Autodesk Fusion 360 part; units mm, degrees
(part 2 of 2)
fillet "Fillet1'" radius 2 5 edges at (-5, 28.7, -10.1) (-4.2678, 59.1678, -10.1) (29, 59.9, -10.1) (62.2678, 59.1678, -10.1) (63, 28.7, -10.1) on bodies 3 in component "versa64case_v2_bottom_closed"
fillet "Fillet5'" radius 0.5 8 edges at (-3, 11.5, -4.85) (-3, 33.3, -4.85) (-3, 35.3, -4.85) (61, 37.9, -4.85) (61, 35.9, -4.85) (61, 11.5, -4.85) (61, 9.5, -4.85) (-3, 9.5, -4.85) on bodies 3 in component "versa64case_v2_bottom_closed"
fillet "Fillet6" radius 0.5 29 edges at (61, 4.5, -8.1) (60.8536, 9.3536, -8.1) (29, 9.5, -8.1) (-2.8536, 9.3536, -8.1) (-3, 4.5, -8.1) (29, 11.5, -8.1) (60.8536, 11.6464, -8.1) (61, 23.7, -8.1) (60.8536, 35.7536, -8.1) (58.5, 35.9, -8.1) (56.1464, 36.0464, -8.1) (56, 36.9, -8.1) (56.1464, 37.7536, -8.1) (58.5, 37.9, -8.1) (60.8536, 38.0464, -8.1) (61, 47.9, -8.1) (60.8536, 57.7536, -8.1) (29, 57.9, -8.1) (-2.8536, 57.7536, -8.1) (-3, 46.6, -8.1) (-2.8536, 35.4464, -8.1) (-0.5, 35.3, -8.1) (1.8536, 35.1536, -8.1) (2, 34.3, -8.1) (1.8536, 33.4464, -8.1) (-0.5, 33.3, -8.1) (-2.8536, 33.1536, -8.1) (-3, 22.4, -8.1) (-2.8536, 11.6464, -8.1) on bodies 3 in component "versa64case_v2_bottom_closed"
fillet "Fillet7'" radius 0.5 6 edges at (25, 47.3, -8.1) (25.1464, 51.0536, -8.1) (29, 51.2, -8.1) (32.8536, 51.0536, -8.1) (33, 47.3, -8.1) (29, 39.9, -8.1) on bodies 3 in component "versa64case_v2_bottom_closed"
chamfer "Chamfer3" distance 2 angle 45 1 edges at (30.4917, 44.4786, -10.1) on bodies 3 in component "versa64case_v2_bottom_closed"
fillet "Fillet8'" radius 0.5 10 edges at (-5, 0, -3.85) (-4.4142, 0, -9.5142) (29, 0, -10.1) (62.4142, 0, -9.5142) (63, 0, -3.85) (61, 0, -4.6) (60.8536, 0, -7.9536) (29, 0, -8.1) (-2.8536, 0, -7.9536) (-3, 0, -4.6) on bodies 3 in component "versa64case_v2_bottom_closed"
fillet "Fillet9" radius 0.5 16 edges at (5, 50.05, -8.1) (5.1464, 52.0536, -8.1) (9, 52.2, -8.1) (12.8536, 52.0536, -8.1) (13, 50.05, -8.1) (12.8536, 48.0464, -8.1) (9, 47.9, -8.1) (5.1464, 48.0464, -8.1) (45, 50.05, -8.1) (45.1464, 52.0536, -8.1) (49, 52.2, -8.1) (52.8536, 52.0536, -8.1) (53, 50.05, -8.1) (52.8536, 48.0464, -8.1) (49, 47.9, -8.1) (45.1464, 48.0464, -8.1) on bodies 3 in component "versa64case_v2_bottom_closed"
fillet "Fillet11" radius 0.5 2 edges at (50.8023, 45.4136, 8.8) (50.8023, 45.4136, 10.8) on bodies 2 in component "Versa64case_v2_top_closed"
sketch "Sketch1 (3)" plane through (0, 0, 10.8) normal (0, 0, 1) x (-1, 0, 0) in component "Label"
  line L0 (3, -0.5) -> (-61, -0.5)
  line L1 (-61, -0.5) -> (-61, -57.4)
  arc A0 (-61, -57.4) -> (-60.5, -57.9) centre (-60.5, -57.4) ccw
  line L2 (-60.5, -57.9) -> (2.5, -57.9)
  arc A1 (2.5, -57.9) -> (3, -57.4) centre (2.5, -57.4) ccw
  line L3 (3, -57.4) -> (3, -0.5)
  circle A2 centre (-52.9, -44.6) radius 2.75
  line L4 (2.5, -57.9) -> (-60.5, -57.9) construction
  arc A3 (2.5, -57.9) -> (3, -57.4) centre (2.5, -57.4) ccw construction
  line L5 (3, -0.5) -> (3, -57.4) construction
  arc A4 (-61, -57.4) -> (-60.5, -57.9) centre (-60.5, -57.4) ccw construction
  line L6 (-61, -57.4) -> (-61, -0.5) construction
  line L7 (-61, -0.5) -> (3, -0.5) construction
  circle A5 centre (-52.9, -44.6) radius 2.75 construction
  line L8 (2.5, -56.9) -> (2.5, -1.5)
  line L9 (2, -1) -> (-60, -1)
  line L10 (-60.5, -1.5) -> (-60.5, -56.9)
  line L11 (-60, -57.4) -> (2, -57.4)
  circle A6 centre (-52.9, -44.6) radius 3.25
  arc A7 (2, -57.4) -> (2.5, -56.9) centre (2, -56.9) ccw
  arc A8 (-60.5, -56.9) -> (-60, -57.4) centre (-60, -56.9) ccw
  arc A9 (-60, -1) -> (-60.5, -1.5) centre (-60, -1.5) ccw
  arc A10 (2.5, -1.5) -> (2, -1) centre (2, -1.5) ccw
  dimension "d231" = 0.5
  dimension "d232" = 0.5
  dimension "d233" = 0.5
  dimension "d234" = 0.5
  dimension "d235" = 0.5
  constraint tangent L8 A7
  constraint tangent L11 A7
  constraint tangent L10 A8
  constraint tangent L11 A8
  constraint tangent L9 A9
  constraint tangent L10 A9
  constraint tangent L8 A10
  constraint tangent L9 A10
  measures "d232" radius of A7
  measures "d233" radius of A8
  measures "d234" radius of A9
  measures "d235" radius of A10
extrude "Extrude1'''" add sketch "Sketch1 (3)" along normal blind 0.1 separate body contours L8 L9 L10 L11 A7 A8 A9 A10 makes body 4 in component "Label"
component "Versa64cart_v1.6" placed x (1, 0, 0) y (0, 1, 0) z (0, 0, 1) at (0, 0, 0)
component "Versa64case_v2_top_closed" placed x (1, 0, 0) y (0, 1, 0) z (0, 0, 1) at (0, 0, 0)
component "versa64case_v2_bottom_closed" placed x (1, 0, 0) y (0, 1, 0) z (0, 0, 1) at (0, 0, 0)
component "Label" placed x (1, 0, 0) y (0, 1, 0) z (0, 0, 1) at (0, 0, 0)
equation "pcb = 1.6 mm"
equation "d2 = -pcb"
equation "d4 = dipsw"
equation "d8 = dipsw + 1.7 mm"
equation "d10 = dipsw - 0.8 mm"
equation "d16 = switch_body"
equation "d18 = switch_body + 0.2 mm"
equation "stem = 12.5 mm"
equation "switch_body = 4.5 mm"
equation "d22 = stem"
equation "dipsw = 5.3 mm"
equation "socket = 4.3 mm"
equation "EPROM = 9.0 mm"
equation "d35 = socket"
equation "d37 = socket"
equation "d38 = EPROM - socket"
equation "above = 8.8 mm"
equation "d42 = above"
equation "below = 6.5 mm"
equation "dside = 3.0 mm"
equation "d45 = dside"
equation "d46 = dside"
equation "dback = 9 mm"
equation "d48 = dback"
equation "ttol = 0.5 mm"
equation "wall = 2 mm"
equation "standoff_top_dia = 6 mm"
equation "d75 = standoff_top_dia"
equation "d76 = ttol"
equation "d77 = ttol"
equation "d78 = ttol"
equation "d79 = ttol"
equation "d80 = ttol"
equation "d81 = ttol"
equation "d82 = ttol"
equation "d83 = ttol"
equation "iwall = 1.2 mm"
equation "portlen = 9.5 mm"
equation "d87 = portlen"
equation "d90 = icorner"
equation "d91 = icorner"
equation "icorner = 0.5 mm"
equation "d93 = swall"
equation "d94 = swall"
equation "d95 = swall"
equation "d96 = icorner + swall"
equation "d97 = icorner + swall"
equation "d98 = wall"
equation "d99 = wall"
equation "d104 = wall"
equation "d105 = wall"
equation "d110 = below"
equation "btol = 0.3 mm"
equation "d114 = btol"
equation "d115 = btol"
equation "standoff_bot_dia = 8 mm"
equation "d117 = standoff_bot_dia"
equation "d119 = btol"
equation "d120 = wall"
equation "d123 = wall"
equation "d125 = btol"
equation "d128 = -above"
equation "d130 = -above"
equation "d134 = -above - pcb"
equation "offset = 2 mm"
equation "d137 = -above - pcb + offset"
equation "d139 = wall / 2"
equation "d141 = btol"
equation "d142 = btol"
equation "d148 = wall"
equation "d150 = -below"
equation "d154 = -below - offset"
equation "d156 = -below - pcb"
equation "d158 = btol"
equation "d159 = btol"
equation "swall = 2.0 mm"
equation "d183 = swall * ofac"
equation "d184 = swall * ofac"
equation "d185 = wall"
equation "d187 = swall * ofac"
equation "d188 = swall * ofac"
equation "d189 = swall * ofac"
equation "d190 = icorner + swall * 0.6"
equation "d191 = icorner + swall * 0.6"
equation "d193 = -below - pcb"
equation "d196 = -below"
equation "d210 = btol"
equation "ofac = 0.43"
equation "d227 = d75 / 2"
equation "d238 = btol"
equation "d239 = btol"
equation "d240 = btol"
equation "d241 = btol"
equation "d242 = btol"
equation "d243 = btol"
equation "d244 = btol"
equation "d245 = btol"
equation "d246 = btol"
equation "d247 = btol"
equation "d248 = btol"
equation "d249 = btol"
named bodies: "versa64cart"
